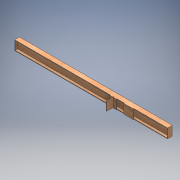
# Autodesk Inventor part: Boom
Saved by Autodesk Inventor 2016 (Build 200138000, 138)
## iProperties
Created: 2016-04-01
Part Number: Boom
Material: Wood (Birch)
Document SubType Name: Modeling
Designer: mkepler
Mass: 193.792 g
Surface Area: 2397.9 cm^2
Volume: 352.35 cm^3
Density: 0.55 g/cm^3
Appearance: Birch - Natural Polished
Author: mkepler
Autodesk Inventor part; units mm, degrees
ref_plane "YZ Plane" through (0, 0, 0) normal (1, 0, 0) x (0, 1, 0)
ref_plane "XZ Plane" through (0, 0, 0) normal (0, 1, 0) x (-1, 0, 0)
ref_plane "XY Plane" through (0, 0, 0) normal (0, 0, 1) x (1, 0, 0)
sketch "Sketch1" plane through (0, 0, 0) normal (0, 1, 0) x (-1, 0, 0)
  line L0 (0, 0) -> (809, 0)
  line L1 (809, 0) -> (809, -50)
  line L2 (809, -50) -> (0, -50)
  line L3 (0, -50) -> (0, 0)
  dimension "d0" = 809
  dimension "d1" = 50
  constraints: 8 end point, 2 parallel, 1 horizontal, 1 perpendicular
  measures "d0" distance of L1.end L2.end
  measures "d1" distance of L0.end L1.end
extrude "Extrusion1" add sketch "Sketch1" along normal blind 3
sketch "Sketch2" plane through (0, 0, 0) normal (0, -1, 0) x (1, 0, 0)
  line L0 (-806, -3) -> (-3, -3)
  line L1 (-3, -3) -> (-3, -47)
  line L2 (-3, -47) -> (-806, -47)
  line L3 (-806, -47) -> (-806, -3)
  line L4 (-809, 0) -> (0, 0) projected
  line L5 (-809, 0) -> (-809, -50) projected
  line L6 (-206, -3) -> (-203, -3)
  line L7 (-203, -3) -> (-203, -47)
  line L8 (-203, -47) -> (-206, -47)
  line L9 (-206, -47) -> (-206, -3)
  line L10 (0, -50) -> (-809, -50) projected
  line L11 (-809, 0) -> (0, 0)
  line L12 (0, 0) -> (0, -50)
  line L13 (0, -50) -> (-809, -50)
  line L14 (-809, -50) -> (-809, 0)
  dimension "d4" = 803
  dimension "d5" = 44
  dimension "d6" = 3
  dimension "d7" = 3
  dimension "d8" = 3
  dimension "d9" = 600
  constraints: 24 end point, 6 parallel, 3 horizontal, 3 perpendicular, 2 point on line
  measures "d4" distance of L1.end L2.end
  measures "d5" distance of L0.end L1.end
  measures "d6" distance between parallel lines of L4 L0
  measures "d7" distance between parallel lines of L5 L3
  measures "d8" distance of L7.end L8.end
  measures "d9" distance between parallel lines of L3 L9
extrude "Extrusion2" add sketch "Sketch2" along normal blind 12.5 and the other way blind 12.5 contours L0 L7 L2 L9 | L4 L12 L10 L5
sketch "Sketch3" plane through (0, -12.5, 0) normal (0, -1, 0) x (1, 0, 0)
  line L0 (0, 0) -> (-809, 0) projected
  line L1 (0, -50) -> (-809, -50) projected
  line L2 (-229.5, 0) -> (-179.5, 0)
  line L3 (-179.5, 0) -> (-179.5, -50)
  line L4 (-179.5, -50) -> (-229.5, -50)
  line L5 (-229.5, -50) -> (-229.5, 0)
  line L6 (-203, -47) -> (-203, -3) projected
  line L7 (-809, 0) -> (0, 0) projected
  line L8 (-269.5, 0) -> (-284.5, 0)
  line L9 (-284.5, 0) -> (-284.5, -50)
  line L10 (-284.5, -50) -> (-269.5, -50)
  line L11 (-269.5, -50) -> (-269.5, 0)
  line L12 (-809, -50) -> (0, -50) projected
  line L13 (-284.5, 0) -> (-287.5, 0)
  line L14 (-287.5, 0) -> (-287.5, -50)
  line L15 (-287.5, -50) -> (-284.5, -50)
  line L16 (-284.5, -50) -> (-284.5, 0)
  line L17 (-287.5, 0) -> (-302.5, 0)
  line L18 (-302.5, 0) -> (-302.5, -50)
  line L19 (-302.5, -50) -> (-287.5, -50)
  line L20 (-287.5, -50) -> (-287.5, 0)
  dimension "d14" = 50
  dimension "d15" = 23.5
  dimension "d18" = 15
  dimension "d19" = 40
  dimension "d24" = 3
  dimension "d25" = 15
  dimension "d26" = 50
  constraints: 32 end point, 8 parallel, 5 point on line, 4 horizontal, 4 perpendicular
  measures "d14" distance of L3.end L4.end
  measures "d15" distance between parallel lines of L6 L3
  measures "d18" distance of L10.end L9.end
  measures "d19" distance between parallel lines of L11 L5
  measures "d24" distance of L15.end L14.end
  measures "d25" distance of L19.end L18.end
  measures "d26" distance between parallel lines of L19 L17
extrude "Extrusion3" add sketch "Sketch3" along normal blind 3 contours L3 L1 L5 L0 | L11 L1 L9 L0 | L14 L1 L18 L0
sketch "Sketch4" plane through (0, 0, 0) normal (0, -1, 0) x (1, 0, 0)
  line L0 (-284.5, -3) -> (-284.5, -47) projected
  line L1 (-284.5, -3) -> (-287.5, -3)
  line L2 (-287.5, -3) -> (-287.5, -47)
  line L3 (-287.5, -47) -> (-284.5, -47)
  line L4 (-284.5, -47) -> (-284.5, -3)
  point P0 (0, 0)
  dimension "d20" = 3
  dimension "d21" = 44
  constraints: 8 end point, 2 parallel, 1 horizontal, 1 perpendicular
  measures "d20" distance of L3.end L2.end
  measures "d21" distance of L2.end L1.end
extrude "Extrusion4" add sketch "Sketch4" along normal blind 50
body "Solid1"
